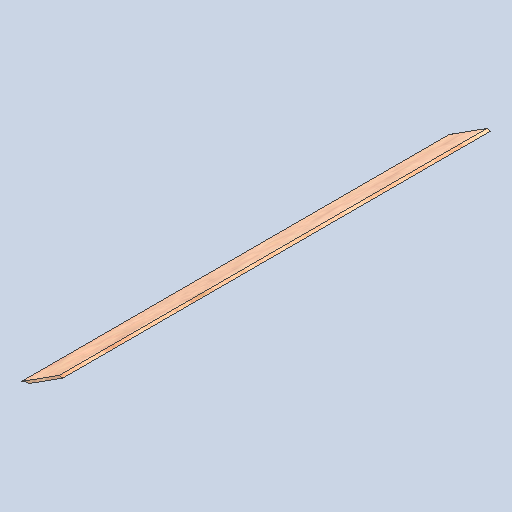
# Autodesk Inventor part: 2P.03.01.06.IM.AileronCutFill
Saved by Autodesk Inventor 2025.2 (Build 292293000, 293)
## iProperties
Created: 2025-01-05
Part Number: 2P.03.01.06.IM.AileronCutFill
Material: Wood (Birch)
Document SubType Name: Modeling
Designer: Imist
Density: 0.55 g/cm^3
Appearance: Birch - Natural Polished
Author: Imist
Autodesk Inventor part; units mm, degrees
ref_plane "YZ Plane" through (0, 0, 0) normal (1, 0, 0) x (0, 1, 0)
ref_plane "XZ Plane" through (0, 0, 0) normal (0, 1, 0) x (-1, 0, 0)
ref_plane "XY Plane" through (0, 0, 0) normal (0, 0, 1) x (1, 0, 0)
sketch "Sketch2" plane through (0, 0, 0) normal (0, 0, 1) x (1, 0, 0)
  line L0 (4.8719, 5.1626) -> (-7.644, -2.8311)
  line L1 (5.3481, 4.5174) -> (-5.1907, -2.2135)
  line L2 (5.3481, 4.5174) -> (6.0672, 4.9767)
  arc A0 (-5.1907, -2.2135) -> (-7.644, -2.8311) centre (-5.4909, -6.2022) ccw
  line L3 (6.0672, 4.9767) -> (4.8719, 5.1626)
  point P0 (5.2456, 5.1046)
  dimension "d8" = 0.8
  dimension "d9" = 8
  constraints: 8 end point, 2 coincident, 2 point on circle, 1 centre point
  measures "d8" distance between parallel lines of L0 L1
  measures "d9" diameter of A0
extrude "Extrusion2" add sketch "Sketch2" along normal blind 142
body "Solid2"
